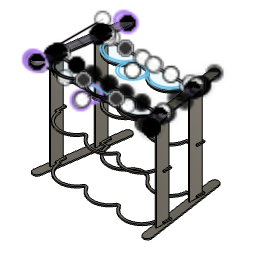
ParametrískurVínrakki (Autodesk Fusion 360 design; units mm, degrees)
Autodesk Fusion 360 part; units mm, degrees
sketch "Sketch2" plane through (0, 0, 0) normal (0, 0, 1) x (1, 0, 0)
  line L0 (0, 0) -> (30, 200)
  line L1 (20.2237, 0) -> (50.2237, 200)
  line L2 (0, 0) -> (80, 0)
  arc A0 (49.865, 201.6378) -> (30, 200) centre (40, 200) ccw
  arc A1 (0, 0) -> (20, 0) centre (10, 0) ccw
  line L3 (29.197, 147.9798) -> (32.197, 147.9798)
  line L4 (32.197, 147.9798) -> (32.197, 135.9798)
  line L5 (32.197, 135.9798) -> (29.197, 135.9798)
  line L6 (29.197, 135.9798) -> (29.197, 147.9798)
  line L7 (15, 100) -> (34.7787, 97.0332)
  line L8 (14.3629, 49.0862) -> (17.3629, 49.0862)
  line L9 (17.3629, 49.0862) -> (17.3629, 37.0862)
  line L10 (17.3629, 37.0862) -> (14.3629, 37.0862)
  line L11 (14.3629, 37.0862) -> (14.3629, 49.0862)
  line L12 (0, 0) -> (300, 0)
  line L13 (150, 0) -> (150, -28.7287)
  arc A2 (270, 200) -> (250.135, 201.6378) centre (260, 200) ccw
  line L14 (285, 100) -> (265.2213, 97.0332)
  line L15 (300, 0) -> (270, 200)
  line L16 (267.803, 147.9798) -> (267.803, 135.9798)
  line L17 (270.803, 147.9798) -> (267.803, 147.9798)
  line L18 (270.803, 135.9798) -> (270.803, 147.9798)
  line L19 (267.803, 135.9798) -> (270.803, 135.9798)
  line L20 (285.6371, 49.0862) -> (282.6371, 49.0862)
  line L21 (282.6371, 37.0862) -> (285.6371, 37.0862)
  line L22 (279.7763, 0) -> (249.7763, 200)
  arc A3 (280, 0) -> (300, 0) centre (290, 0) ccw
  line L23 (285.6371, 37.0862) -> (285.6371, 49.0862)
  line L24 (282.6371, 49.0862) -> (282.6371, 37.0862)
  line L25 (40, 200) -> (10, 0)
  line L26 (49.865, 201.6378) -> (50.2237, 200)
  line L27 (250.135, 201.6378) -> (249.7763, 200)
  point P0 (300, 0)
  point P1 (300, 0)
  point P2 (300, 0)
  dimension "d4" = 20
  dimension "d5" = 200
  dimension "d6" = 200
  dimension "d7" = 30
  dimension "d8" = 10
  dimension "d9" = 10
  dimension "d13" = 3
  dimension "d14" = 12
  dimension "d17" = 3
  dimension "d18" = 50
  dimension "d19" = 12
  dimension "d22" = 300
  dimension "d43" = 50
  constraint coincident L0.start L2.start
  constraint parallel L0 L1
  constraint horizontal L2
  constraint coincident L1.start L2
  constraint coincident L2 A1.centre
  constraint horizontal L3
  constraint vertical L4
  constraint horizontal L5
  constraint vertical L6
  constraint midpoint L0 L7.start
  constraint coincident L1 L7.end
  constraint perpendicular L1 L7
  constraint horizontal L8
  constraint vertical L9
  constraint horizontal L10
  constraint vertical L11
  constraint parallel L2 L12
  constraint midpoint L12 L13.start
  constraint perpendicular L12 L13
  constraint symmetric L0.start L13 P2
  constraint symmetric L0.end L13 A2.start
  constraint symmetric L1.start L13 L22.start
  constraint symmetric L1.end L13 L22.end
  constraint symmetric A0.start L13 A2.end
  constraint symmetric A0 L13 A2
  constraint symmetric A1.end L13 A3.start
  constraint symmetric A1 L13 A3
  constraint symmetric L3.start L13 L17.start
  constraint symmetric L3.end L13 L16.start
  constraint symmetric L4.end L13 L16.end
  constraint symmetric L5.end L13 L18.start
  constraint symmetric L7.start L13 L14.start
  constraint symmetric L7.end L13 L14.end
  constraint symmetric L8.start L13 L20.start
  constraint symmetric L8.end L13 L20.end
  constraint symmetric L9.end L13 L21.start
  constraint symmetric L10.end L13 L21.end
  constraint coincident A0.centre L25.start
  constraint coincident A1.centre L25.end
  constraint parallel L1 L25
  constraint coincident L8.end L25
  constraint coincident L3.end L25
  measures "d4" distance of L0 L1
  measures "d5" vertical distance of L0.start L0.end
  measures "d6" vertical distance of L0.start L1.end
  measures "d7" horizontal distance of L0.start L0.end
  measures "d8" radius of A1
  measures "d9" radius of A0
  measures "d13" distance of L4 L6
  measures "d14" distance of L3 L5
  measures "d17" distance of L9 L11
  measures "d18" distance of L7 L8.end
  measures "d19" distance of L8.end L9.end
  measures "d22" distance of L0.start P2
  measures "d43" distance of L3.end L7
sketch "Sketch3" plane through (0, 0, 0) normal (0, 0, 1) x (1, 0, 0)
  line L0 (14.3629, 49.0862) -> (17.3629, 49.0862)
  line L1 (17.3629, 49.0862) -> (17.3629, 37.0862)
  line L2 (14.3629, 37.0862) -> (14.3629, 49.0862)
  line L3 (17.3629, 37.0862) -> (14.3629, 37.0862)
  line L4 (32.197, 147.9798) -> (32.197, 135.9798)
  line L5 (29.197, 135.9798) -> (29.197, 147.9798)
  line L6 (29.197, 147.9798) -> (32.197, 147.9798)
  line L7 (32.197, 135.9798) -> (29.197, 135.9798)
  line L8 (270.803, 135.9798) -> (270.803, 147.9798)
  line L9 (267.803, 147.9798) -> (267.803, 135.9798)
  line L10 (270.803, 147.9798) -> (267.803, 147.9798)
  line L11 (267.803, 135.9798) -> (270.803, 135.9798)
  line L12 (285.6371, 49.0862) -> (282.6371, 49.0862)
  line L13 (285.6371, 37.0862) -> (285.6371, 49.0862)
  line L14 (282.6371, 49.0862) -> (282.6371, 37.0862)
  line L15 (282.6371, 37.0862) -> (285.6371, 37.0862)
  line L16 (0, 0) -> (300, 0)
  line L17 (150, 0) -> (150, -24.5455)
  line L18 (29.197, 141.9798) -> (25.697, 141.9798)
  line L19 (25.697, 141.9798) -> (25.697, 151.4798)
  line L20 (25.697, 151.4798) -> (37.197, 151.4798)
  line L21 (37.197, 151.4798) -> (37.197, 141.9798)
  line L22 (22.3629, 43.0862) -> (22.3629, 52.5862)
  line L23 (22.3629, 52.5862) -> (10.8629, 52.5862)
  line L24 (10.8629, 52.5862) -> (10.8629, 43.0862)
  line L25 (10.8629, 43.0862) -> (14.3629, 43.0862)
  line L26 (274.303, 141.9798) -> (274.303, 151.4798)
  line L27 (274.303, 151.4798) -> (262.803, 151.4798)
  line L28 (262.803, 151.4798) -> (262.803, 141.9798)
  line L29 (277.6371, 52.5862) -> (289.1371, 52.5862)
  line L30 (277.6371, 43.0862) -> (277.6371, 52.5862)
  line L31 (289.1371, 52.5862) -> (289.1371, 43.0862)
  line L32 (289.1371, 43.0862) -> (285.6371, 43.0862)
  line L33 (270.803, 141.9798) -> (274.303, 141.9798)
  line L34 (0, 0) -> (0, 176.4903)
  line L35 (40, 200) -> (10, 0)
  line L36 (17.3629, 37.0862) -> (16.6076, 0)
  line L37 (0, 0) -> (30, 200)
  line L38 (0, 0) -> (9.7217, -1.4583)
  line L39 (29.197, 147.9798) -> (22.197, 147.9798)
  line L40 (32.197, 147.9798) -> (52, 147.9798)
  line L41 (37.197, 141.9798) -> (262.803, 141.9798)
  line L42 (32.197, 136.9798) -> (267.803, 136.9798)
  arc A0 (52.197, 141.9798) -> (132.1968, 141.8687) centre (92.197, 141.9798) ccw
  arc A1 (47.197, 141.9798) -> (137.1968, 141.8549) centre (92.197, 141.9798) ccw
  arc A2 (167.5793, 141.9798) -> (247.5791, 141.8687) centre (207.5793, 141.9798) ccw
  arc A3 (162.5793, 141.9798) -> (252.5791, 141.8549) centre (207.5793, 141.9798) ccw
  line L43 (22.3629, 43.0862) -> (277.6371, 43.0862)
  line L44 (17.3629, 38.0862) -> (282.6371, 38.0862)
  arc A4 (27.3629, 43.0862) -> (107.3622, 42.8457) centre (67.3629, 43.0862) ccw
  arc A5 (22.3629, 43.0862) -> (112.3621, 42.8156) centre (67.3629, 43.0862) ccw
  circle A6 centre (149.8881, 102.4129) radius 29.9558
  circle A7 centre (149.8881, 102.4129) radius 24.9558
  arc A8 (105, 43.0862) -> (194.9992, 42.8156) centre (150, 43.0862) ccw
  arc A9 (110, 43.0862) -> (189.9993, 42.8457) centre (150, 43.0862) ccw
  arc A10 (187.6371, 43.0862) -> (277.6363, 42.8156) centre (232.6371, 43.0862) ccw
  arc A11 (192.6371, 43.0862) -> (272.6363, 42.8457) centre (232.6371, 43.0862) ccw
  circle A12 centre (108.6815, 19.5466) radius 7.5535
  circle A13 centre (108.6815, 19.5466) radius 2.5535
  line L45 (108.6815, 19.5466) -> (220, 19.5466)
  circle A14 centre (191.3185, 19.5466) radius 7.5535
  circle A15 centre (191.3185, 19.5466) radius 2.5535
  line L46 (112.3621, 42.8156) -> (112.3637, 43.0862)
  line L47 (107.3622, 42.8457) -> (107.3637, 43.0862)
  line L48 (194.9992, 42.8156) -> (195.0008, 43.0862)
  line L49 (189.9993, 42.8457) -> (190.0007, 43.0862)
  line L50 (272.6363, 42.8457) -> (272.6378, 43.0862)
  line L51 (277.6363, 42.8156) -> (277.6371, 43.0862)
  line L52 (247.5791, 141.8687) -> (247.5794, 141.9798)
  line L53 (252.5791, 141.8549) -> (252.5795, 141.9798)
  line L54 (25.697, 151.4798) -> (25.697, 161.4798)
  line L55 (25.697, 161.4798) -> (37.197, 161.4798)
  line L56 (37.197, 161.4798) -> (37.197, 151.4798)
  line L57 (10.8629, 52.5862) -> (10.8629, 62.5862)
  line L58 (10.8629, 62.5862) -> (22.3629, 62.5862)
  line L59 (22.3629, 62.5862) -> (22.3629, 52.5862)
  line L60 (29.197, 147.9798) -> (29.197, 157.9798)
  line L61 (29.197, 157.9798) -> (32.197, 157.9798)
  line L62 (32.197, 157.9798) -> (32.197, 147.9798)
  line L63 (14.3629, 49.0862) -> (14.3629, 59.0862)
  line L64 (14.3629, 59.0862) -> (17.3629, 59.0862)
  line L65 (17.3629, 59.0862) -> (17.3629, 49.0862)
  line L66 (285.6371, 49.0862) -> (285.6371, 59.0862)
  line L67 (282.6371, 59.0862) -> (282.6371, 49.0862)
  line L68 (285.6371, 59.0862) -> (282.6371, 59.0862)
  line L69 (289.1371, 52.5862) -> (289.1371, 62.5862)
  line L70 (289.1371, 62.5862) -> (277.6371, 62.5862)
  line L71 (277.6371, 62.5862) -> (277.6371, 52.5862)
  line L72 (270.803, 147.9798) -> (270.803, 157.9798)
  line L73 (267.803, 157.9798) -> (267.803, 147.9798)
  line L74 (274.303, 151.4798) -> (274.303, 161.4798)
  line L75 (274.303, 161.4798) -> (262.803, 161.4798)
  line L76 (262.803, 161.4798) -> (262.803, 151.4798)
  line L77 (270.803, 157.9798) -> (267.803, 157.9798)
  dimension "d25" = 300
  dimension "d26" = 3.5
  dimension "d27" = 3.5
  dimension "d29" = 3.5
  dimension "d30" = 3.5
  dimension "d31" = 5
  dimension "d33" = 5
  dimension "d37" = 90
  dimension "d46" = 5
  dimension "d47" = 9.5
  dimension "d48" = 40
  dimension "d49" = 5
  dimension "d51" = 10
  dimension "d54" = 115.3823
  dimension "d55" = 0
  dimension "d56" = 9.5
  dimension "d57" = 5
  dimension "d58" = 5
  dimension "d60" = 40
  dimension "d70" = 165.2741
  dimension "d71" = 0
  dimension "d98" = 11.5
  dimension "d99" = 11.5
  dimension "d100" = 10
  dimension "d101" = 10
  dimension "d102" = 3
  dimension "d103" = 10
  dimension "d104" = 3
  dimension "d105" = 10
  constraint coincident L16.start L34.start
  constraint perpendicular L4 L16
  constraint midpoint L16 L17.start
  constraint perpendicular L16 L17
  constraint midpoint L5 L18.start
  constraint perpendicular L5 L18
  constraint perpendicular L18 L19
  constraint perpendicular L19 L20
  constraint perpendicular L20 L21
  constraint parallel L2 L22
  constraint perpendicular L22 L23
  constraint perpendicular L23 L24
  constraint midpoint L2 L25.end
  constraint perpendicular L2 L25
  constraint symmetric L17 L18.start L33.start
  constraint symmetric L17 L18.end L26.start
  constraint symmetric L17 L19.end L26.end
  constraint symmetric L17 L20.end L27.end
  constraint symmetric L17 L21.end L28.end
  constraint symmetric L17 L22.start L30.start
  constraint symmetric L17 L22.end L29.start
  constraint symmetric L17 L23.end L29.end
  constraint symmetric L17 L24.end L31.end
  constraint symmetric L17 L25.end L32.end
  constraint perpendicular L16 L34
  constraint coincident L1.end L3.start
  constraint coincident L16 L36.end
  constraint coincident L5.end L6.start
  constraint coincident L37 L39.end
  constraint perpendicular L19 L39
  constraint coincident L4.start L6.end
  constraint perpendicular L4 L40
  constraint coincident L4 L42.start
  constraint coincident L9 L42.end
  constraint perpendicular L9 L42
  constraint coincident L41 A0.start
  constraint coincident L41 A0.centre
  constraint coincident L1 L44.start
  constraint coincident L14 L44.end
  constraint perpendicular L14 L44
  constraint coincident L43 A4.start
  constraint coincident L43 A4.centre
  constraint tangent A2 A6
  constraint tangent A0 A6
  constraint concentric A6 A7
  constraint tangent A3 A7
  constraint coincident L22.start L43.start
  constraint tangent A9 A12
  constraint tangent A4 A12
  constraint concentric A12 A13
  constraint tangent A8 A13
  constraint coincident A12.centre A13.centre
  constraint horizontal L45
  constraint coincident L45 A14.centre
  constraint tangent A11 A14
  constraint tangent A9 A14
  constraint concentric A14 A15
  constraint tangent A10 A15
  constraint coincident L43 L46.end
  constraint tangent A5 L46
  constraint coincident L43 L47.end
  constraint tangent A4 L47
  constraint coincident L43 L48.end
  constraint tangent A8 L48
  constraint coincident L43 L49.end
  constraint tangent A9 L49
  constraint parallel L48 L49
  constraint coincident L43 L50.end
  constraint tangent A11 L50
  constraint coincident L41 L52.end
  constraint tangent A2 L52
  constraint coincident L41 L53.end
  constraint tangent A3 L53
  constraint parallel L52 L53
  constraint perpendicular L20 L54
  constraint perpendicular L19 L55
  constraint perpendicular L20 L56
  constraint perpendicular L23 L57
  constraint perpendicular L24 L58
  constraint perpendicular L58 L59
  constraint perpendicular L39 L60
  constraint perpendicular L5 L61
  constraint coincident L40 L4.start
  constraint perpendicular L40 L62
  constraint coincident L0.start L2.end
  constraint perpendicular L23 L63
  constraint perpendicular L2 L64
  constraint perpendicular L23 L65
  constraint symmetric L17 L54.end L74.end
  constraint symmetric L17 L55.end L75.end
  constraint symmetric L17 L57.end L69.end
  constraint symmetric L17 L58.end L70.end
  constraint symmetric L17 L5.end L8.end
  constraint symmetric L17 L60.end L72.end
  constraint symmetric L17 L61.end L73.start
  constraint symmetric L17 L4.start L9.start
  constraint symmetric L17 L0.start L12.start
  constraint symmetric L17 L63.end L66.end
  constraint symmetric L17 L64.end L67.start
  constraint symmetric L17 L0.end L12.end
  measures "d25" distance of L16.start L16.end
  measures "d26" distance of L5 L19
  measures "d27" distance of L6 L20
  measures "d29" distance of L2 L24
  measures "d30" distance of L0 L23
  measures "d31" distance of L1 L22
  measures "d33" distance of L4 L21
  measures "d37" angle of L37 L38
  measures "d46" distance of L41 L42
  measures "d47" distance of L20 L21.end
  measures "d48" radius of A0
  measures "d51" distance of L21.end A1.start
  measures "d56" distance of L22.start L22.end
  measures "d57" distance of L43 L44
  measures "d60" radius of A4
  measures "d98" distance of L54 L56
  measures "d99" distance of L57 L59
  measures "d100" distance of L23 L58
  measures "d101" distance of L20 L55
  measures "d102" distance of L60 L62
  measures "d103" distance of L6 L61
  measures "d104" distance of L63 L65
  measures "d105" distance of L0 L64
extrude "Extrude1" add sketch "Sketch2" along normal blind 3 contours L0 L2 L7 L8 L10 L11 L12 L25 | L2 A1 L12 | L0 L1 A0 L7 L26 | L1 L2 L7 L9 L10 L12 L25 | L12 L14 L15 L22 | L12 A3 | A2 L14 L15 L22 L27 makes body 1 at (37.4736, 182.6599, 0) makes body 2 at (262.5264, 182.6599, 0)
sketch "Sketch4" plane through (0, 0, 0) normal (0, 0, 1) x (1, 0, 0)
  line L0 (29.197, 135.9798) -> (29.197, 147.9798)
  line L1 (32.197, 147.9798) -> (32.197, 135.9798)
  line L2 (29.197, 147.9798) -> (32.197, 147.9798)
  line L3 (32.197, 135.9798) -> (29.197, 135.9798)
  line L4 (150, 0) -> (150, -28.7287)
  line L5 (17.3629, 49.0862) -> (17.3629, 37.0862)
  line L6 (14.3629, 37.0862) -> (14.3629, 49.0862)
  line L7 (14.3629, 49.0862) -> (17.3629, 49.0862)
  line L8 (17.3629, 37.0862) -> (14.3629, 37.0862)
  line L9 (29.197, 147.9798) -> (29.197, 157.9798)
  line L10 (29.197, 157.9798) -> (32.197, 157.9798)
  line L11 (32.197, 157.9798) -> (32.197, 146.8117)
  line L12 (29.197, 135.9798) -> (29.197, 125.9798)
  line L13 (29.197, 125.9798) -> (32.197, 125.9798)
  line L14 (32.197, 125.9798) -> (32.197, 139.521)
  line L15 (14.3629, 49.0862) -> (14.3629, 59.0862)
  line L16 (14.3629, 59.0862) -> (17.3629, 59.0862)
  line L17 (17.3629, 59.0862) -> (17.3629, 49.0862)
  line L18 (14.3629, 37.0862) -> (14.3629, 27.0862)
  line L19 (14.3629, 27.0862) -> (17.3629, 27.0862)
  line L20 (17.3629, 27.0862) -> (17.3629, 37.0862)
  line L21 (285.6371, 49.0862) -> (285.6371, 59.0862)
  line L22 (285.6371, 59.0862) -> (282.6371, 59.0862)
  line L23 (282.6371, 59.0862) -> (282.6371, 49.0862)
  line L24 (285.6371, 37.0862) -> (285.6371, 27.0862)
  line L25 (285.6371, 27.0862) -> (282.6371, 27.0862)
  line L26 (282.6371, 27.0862) -> (282.6371, 37.0862)
  line L27 (270.803, 135.9798) -> (270.803, 125.9798)
  line L28 (270.803, 125.9798) -> (267.803, 125.9798)
  line L29 (267.803, 125.9798) -> (267.803, 139.521)
  line L30 (267.803, 157.9798) -> (267.803, 146.8117)
  line L31 (270.803, 157.9798) -> (267.803, 157.9798)
  line L32 (270.803, 147.9798) -> (270.803, 157.9798)
  line L33 (282.6371, 49.0862) -> (285.6371, 49.0862)
  line L34 (285.6371, 37.0862) -> (280, 37.0862)
  line L35 (270.803, 135.9798) -> (255, 135.9798)
  line L36 (270.803, 147.9798) -> (251, 147.9798)
  dimension "d79" = 3
  dimension "d80" = 10
  dimension "d81" = 3
  dimension "d82" = 10
  dimension "d83" = 3
  dimension "d84" = 10
  dimension "d85" = 3
  dimension "d86" = 10
  constraint coincident L0.end L2.start
  constraint perpendicular L2 L9
  constraint perpendicular L9 L10
  constraint perpendicular L10 L11
  constraint coincident L0.start L3.end
  constraint perpendicular L3 L12
  constraint perpendicular L12 L13
  constraint perpendicular L13 L14
  constraint coincident L6.end L7.start
  constraint perpendicular L7 L15
  constraint perpendicular L15 L16
  constraint perpendicular L16 L17
  constraint coincident L6.start L8.end
  constraint perpendicular L8 L18
  constraint perpendicular L18 L19
  constraint perpendicular L8 L20
  constraint symmetric L4 L0.end L32.start
  constraint symmetric L4 L9.end L31.start
  constraint symmetric L4 L10.end L30.start
  constraint symmetric L4 L11.end L30.end
  constraint symmetric L4 L0.start L27.start
  constraint symmetric L4 L12.end L27.end
  constraint symmetric L4 L13.end L28.end
  constraint symmetric L4 L14.end L29.end
  constraint symmetric L4 L6.end L21.start
  constraint symmetric L4 L15.end L21.end
  constraint symmetric L4 L16.end L22.end
  constraint symmetric L4 L5.start L23.end
  constraint symmetric L4 L6.start L24.start
  constraint symmetric L4 L18.end L24.end
  constraint symmetric L4 L19.end L25.end
  constraint symmetric L4 L5.end L26.end
  constraint coincident L5.start L7.end
  constraint perpendicular L26 L34
  constraint coincident L26.end L34
  constraint perpendicular L27 L35
  constraint perpendicular L32 L36
  measures "d79" distance of L9 L11
  measures "d80" distance of L2 L10
  measures "d81" distance of L12 L14
  measures "d82" distance of L3 L13
  measures "d83" distance of L18 L20
  measures "d84" distance of L8 L19
  measures "d85" distance of L15 L17
  measures "d86" distance of L7 L16
extrude "Extrude4" add sketch "Sketch2" along normal blind 3 from surface at -244 separate body contours L0 L2 L7 L8 L10 L11 L12 L25 | L2 A1 L12 | L0 L1 A0 L7 L26 | L1 L2 L7 L9 L10 L12 L25 | L12 L14 L15 L22 | L12 A3 | A2 L14 L15 L22 L27 makes body 3 at (37.4736, 182.6599, -244) makes body 4 at (262.5264, 182.6599, -244)
extrude "Extrude5" add sketch "Sketch2" sketch "Sketch4" against normal blind 241 separate body contours L16 L17 L18 L19 | L20 L21 L23 L24 of sketch 2 makes body 5 at (17.3629, 48.4195, -80.3333) makes body 6 at (270.803, 136.6465, -80.3333) makes body 7 at (285.6371, 37.7529, -80.3333) makes body 8 at (29.197, 136.6465, -80.3333)
extrude "Extrude6" add sketch "Sketch2" along normal blind 3 contours L9 L10 L25 | L8 L10 L11 L25 | L3 L5 L6 L25 | L4 L5 L25 | L16 L17 L18 L19 | L20 L21 L23 L24 bodies 5 6 7 8
extrude "Extrude7" add sketch "Sketch2" along normal blind 3 from surface at -244 contours L9 L10 L25 | L8 L10 L11 L25 | L3 L5 L6 L25 | L4 L5 L25 | L16 L17 L18 L19 | L20 L21 L23 L24 bodies 5 6 7 8
extrude "Extrude8" add sketch "Sketch3" along normal blind 3 from surface at -238 separate body contours L2 L23 L24 L25 L63 | L1 L22 L23 L35 L44 A5 | L23 L35 L65 | L23 L35 L57 L58 L63 L64 L65 | L23 L35 L58 L59 | L43 L44 A4 A5 | L16 L44 A4 A5 A12 | L16 A5 | A5 A8 A12 | L4 L21 L40 L41 L42 A1 | L20 L35 L62 | L20 L21 L35 L40 | A5 A8 A12 | L16 A8 A9 A12 L45 A14 | L16 L17 A8 | L5 L18 L19 L39 | L19 L20 L39 L60 | L20 L35 L55 L56 | L20 L35 L54 L55 L60 L61 L62 | A5 A8 A13 | A5 A8 A12 L45 | A8 A12 L45 | L16 L17 A8 | L41 L42 A0 A1 | L42 A0 A1 A6 | A9 A12 L45 | A1 A6 | L16 L44 A10 A11 L45 A14 | L16 A10 | A8 L45 A14 | A1 A3 A6 A7 | A9 L45 A14 | A10 L45 A14 | A8 A10 L45 A14 | A3 A6 | L42 A2 A3 A6 | A8 A10 A14 | L14 L29 L30 L44 A10 L51 L67 | L43 L44 A10 A11 L50 L51 | A8 A10 L45 A14 | A11 L45 A14 | A8 A10 A15 | L9 L27 L28 L41 L42 A3 L53 L73 | L41 L42 A2 A3 L52 L53 | L13 L29 L31 L32 L66 | L29 L66 L67 L68 L69 L70 L71 | L8 L26 L27 L33 L72 | L27 L72 L73 L74 L75 L76 L77 picked at (49.5406, 134.8843) picked at (161.4341, 128.164) picked at (250.2357, 134.8843) makes body 9 at (33.8636, 145.6465, -235) makes body 10 at (19.0296, 46.7529, -238)
extrude "Extrude9" add sketch "Sketch3" along normal blind 3 from surface at -125 separate body contours L2 L23 L24 L25 L63 | L1 L22 L23 L35 L44 A5 | L23 L35 L57 L58 L63 L64 L65 | L23 L35 L58 L59 | L43 L44 A4 A5 | L16 L44 A4 A5 A12 | L16 A5 | A5 A8 A12 | L4 L21 L40 L41 L42 A1 | L20 L21 L35 L40 | A5 A8 A12 | L16 A8 A9 A12 L45 A14 | L16 L17 A8 | L5 L18 L19 L39 | L19 L20 L39 L60 | L20 L35 L55 L56 | L20 L35 L54 L55 L60 L61 L62 | A5 A8 A13 | A5 A8 A12 L45 | A8 A12 L45 | L16 L17 A8 | L41 L42 A0 A1 | L42 A0 A1 A6 | A9 A12 L45 | A1 A6 | L16 L44 A10 A11 L45 A14 | L16 A10 | A8 L45 A14 | A1 A3 A6 A7 | A9 L45 A14 | A10 L45 A14 | A8 A10 L45 A14 | A3 A6 | L42 A2 A3 A6 | A8 A10 A14 | L14 L29 L30 L44 A10 L51 L67 | L43 L44 A10 A11 L50 L51 | A8 A10 L45 A14 | A11 L45 A14 | A8 A10 A15 | L9 L27 L28 L41 L42 A3 L53 L73 | L41 L42 A2 A3 L52 L53 | L13 L29 L31 L32 L66 | L29 L66 L67 L68 L69 L70 L71 | L8 L26 L27 L33 L72 | L27 L72 L73 L74 L75 L76 L77 picked at (49.5406, 134.8843) picked at (161.4341, 128.164) picked at (250.2357, 134.8843) makes body 11 at (266.1364, 145.6465, -125) makes body 12 at (280.9704, 46.7529, -125)
extrude "Extrude10" add sketch "Sketch3" along normal blind 3 from surface at -9 separate body contours L2 L23 L24 L25 L63 | L1 L22 L23 L35 L44 A5 | L23 L35 L65 | L23 L35 L57 L58 L63 L64 L65 | L23 L35 L58 L59 | L43 L44 A4 A5 | L16 L44 A4 A5 A12 | L16 A5 | A5 A8 A12 | L4 L21 L40 L41 L42 A1 | L20 L35 L62 | L20 L21 L35 L40 | A5 A8 A12 | L16 A8 A9 A12 L45 A14 | L16 L17 A8 | L5 L18 L19 L39 | L19 L20 L39 L60 | L20 L35 L55 L56 | L20 L35 L54 L55 L60 L61 L62 | A5 A8 A13 | A5 A8 A12 L45 | A8 A12 L45 | L16 L17 A8 | L41 L42 A0 A1 | L42 A0 A1 A6 | A9 A12 L45 | A1 A6 | L16 L44 A10 A11 L45 A14 | L16 A10 | A8 L45 A14 | A1 A3 A6 A7 | A9 L45 A14 | A10 L45 A14 | A8 A10 L45 A14 | A3 A6 | L42 A2 A3 A6 | A8 A10 A14 | L14 L29 L30 L44 A10 L51 L67 | L43 L44 A10 A11 L50 L51 | A8 A10 L45 A14 | A11 L45 A14 | A8 A10 A15 | L9 L27 L28 L41 L42 A3 L53 L73 | L41 L42 A2 A3 L52 L53 | L13 L29 L31 L32 L66 | L29 L66 L67 L68 L69 L70 L71 | L8 L26 L27 L33 L72 | L27 L72 L73 L74 L75 L76 L77 picked at (49.5406, 134.8843) picked at (161.4341, 128.164) picked at (250.2357, 134.8843) makes body 13 at (33.8636, 145.6465, -6) makes body 14 at (19.0296, 46.7529, -9)
equation "hæðstyrkingu = 200 mm"
equation "breiddstyrkingu = 30 mm"
equation "þykktStyrkingu = 20 mm"
equation "d4 = þykktStyrkingu"
equation "d5 = hæðstyrkingu"
equation "d6 = hæðstyrkingu"
equation "d7 = breiddstyrkingu"
equation "d8 = þykktStyrkingu / 2"
equation "d9 = þykktStyrkingu / 2"
equation "efni = 3 mm"
equation "fingur1 = 12 mm"
equation "ofset = hæðstyrkingu / 4"
equation "d13 = efni"
equation "d14 = fingur1"
equation "d17 = efni"
equation "d18 = ofset"
equation "d19 = fingur1"
equation "lengdRakka = 300 mm"
equation "d22 = lengdRakka"
equation "avgD = 80 mm"
equation "breidd = 250 mm"
equation "d25 = lengdRakka"
equation "d26 = efni + 0.5 mm"
equation "d27 = efni + 0.5 mm"
equation "d29 = efni + 0.5 mm"
equation "d30 = efni + 0.5 mm"
equation "d31 = þykktStyrkingu / 4"
equation "d33 = þykktStyrkingu / 4"
equation "bilid = þykktStyrkingu / 4 + þykktStyrkingu / 2 + ( ( L_skálína ) / 2 - L_vantar - ofset ) * cos(v)"
equation "v = atan(hæðstyrkingu / breiddstyrkingu)"
equation "L_skálína = sqrt(hæðstyrkingu ^ 2 + breiddstyrkingu ^ 2)"
equation "w = 90 deg - v"
equation "L_vantar = sin(w) * þykktStyrkingu / 2"
equation "bil_niðri = lengdRakka - bilid * 2"
equation "bilid2 = ( okihvaðeraðfrettaher + þykktStyrkingu / 4 ) + k"
equation "k = ( ( L_skálína / 2 - L_vantar + ofset ) ) * sin(w)"
equation "d43 = ofset"
equation "bil_uppi = lengdRakka - 2 * bilid2"
equation "okihvaðeraðfrettaher = ( þykktStyrkingu / 2 ) / cos(w)"
equation "d46 = þykktStyrkingu / 4"
equation "d47 = fingur1 / 2 + efni + 0.5 mm"
equation "d48 = avgD / 2"
equation "d49 = þykktStyrkingu / 4"
equation "ofset_hringur = 10 mm"
equation "d51 = ofset_hringur"
equation "d54 = bil_uppi - ( avgD + þykktStyrkingu / 2 + ofset_hringur * 2 )"
equation "d56 = fingur1 / 2 + efni + 0.5 mm"
equation "d57 = þykktStyrkingu / 4"
equation "d58 = þykktStyrkingu / 4"
equation "d60 = avgD / 2"
equation "ofset_hringur_niðri = 0 mm"
equation "d70 = bil_niðri - ( avgD + þykktStyrkingu / 2 )"
equation "d72 = efni"
equation "d79 = efni"
equation "d80 = þykktStyrkingu / 2"
equation "d81 = efni"
equation "d82 = þykktStyrkingu / 2"
equation "d83 = efni"
equation "d84 = þykktStyrkingu / 2"
equation "d85 = efni"
equation "d86 = þykktStyrkingu / 2"
equation "d87 = -breidd + efni * 2"
equation "d88 = efni"
equation "d90 = -breidd + efni * 3"
equation "d92 = efni"
equation "d94 = -breidd + efni * 2"
equation "d95 = efni"
equation "d98 = þykktStyrkingu / 4 + efni * 2 + 0.5 mm"
equation "d99 = þykktStyrkingu / 4 + efni * 2 + 0.5 mm"
equation "d100 = þykktStyrkingu / 2"
equation "d101 = þykktStyrkingu / 2"
equation "d102 = efni"
equation "d103 = þykktStyrkingu / 2"
equation "d104 = efni"
equation "d105 = þykktStyrkingu / 2"
equation "d106 = -breidd + 4 * efni"
equation "d107 = efni"
equation "d109 = -breidd / 2"
equation "d110 = efni"
equation "d112 = -3 * efni"
equation "d113 = efni"
